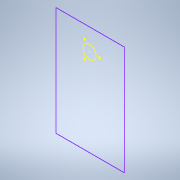
# Autodesk Inventor part: Linker_Structure
Saved by Autodesk Inventor 2020 (Build 240168000, 168)
## iProperties
Created: 2021-06-11
Part Number: Linker_Structure
Material: 一般
Document SubType Name: Modeling
Designer: user
Density: 1 g/cm^3
Appearance: 預設
Author: user
Autodesk Inventor part; units mm, degrees
ref_plane "YZ Plane" through (0, 0, 0) normal (1, 0, 0) x (0, 1, 0)
ref_plane "XZ Plane" through (0, 0, 0) normal (0, 1, 0) x (-1, 0, 0)
ref_plane "XY Plane" through (0, 0, 0) normal (0, 0, 1) x (1, 0, 0)
sketch "草圖1" plane through (0, 0, 0) normal (0, 0, 1) x (1, 0, 0)
  circle A0 centre (15, 0) radius 1.5 projected
  circle A1 centre (-7.5, -12.9904) radius 1.5 projected
  circle A2 centre (-7.5, 12.9904) radius 1.5 projected
  circle A3 centre (0, 0) radius 9.94 projected
  arc A4 (24.2558, 6.0545) -> (-24.6882, 3.9362) centre (0, 0) ccw
  arc A5 (-25.4732, -69.9345) -> (3.0268, -98.4345) centre (3.0268, -69.9345) ccw projected
  arc A6 (3.0268, -98.4345) -> (31.5268, -69.9345) centre (3.0268, -69.9345) ccw projected
  arc A7 (-35.4868, -63.7941) -> (40.8658, -60.4896) centre (3.0268, -69.9345) ccw
  line L0 (24.2558, 6.0545) -> (40.8658, -60.4896)
  line L1 (-24.6882, 3.9362) -> (-35.4868, -63.7941)
  circle A8 centre (26.5268, -93.4345) radius 2.5 projected
  circle A9 centre (-20.4732, -93.4345) radius 2.5 projected
  circle A10 centre (-20.4732, -46.4345) radius 2.5 projected
  circle A11 centre (26.5268, -46.4345) radius 2.5 projected
  circle A12 centre (3.0268, -69.9345) radius 19 projected
  circle A13 centre (3.0268, -69.9345) radius 19.5
  circle A14 centre (0, 0) radius 10.5
  point P0 (0, 0)
  dimension "d1" = 50
  dimension "d2" = 78
  dimension "d3" = 39
  dimension "d4" = 21
  constraints: 4 centre point, 4 coincident, 4 end point, 4 point on circle, 4 tangent
  measures "d1" diameter of A4
  measures "d2" diameter of A7
  measures "d3" diameter of A13
  measures "d4" diameter of A14
extrude "擠出1" add sketch "草圖1" along normal blind 4 contours L0 A7 L1 A4
